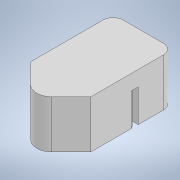
# Autodesk Inventor part: Belt Clip
Saved by Autodesk Inventor 2022 (Build 260153000, 153)
## iProperties
Created: 2022-06-13
Part Number: Belt Clip
Material: Generic
Document SubType Name: Modeling
Designer: Nick
Density: 1 g/cm^3
Appearance: Default
Author: Nick
Autodesk Inventor part; units mm, degrees
ref_plane "YZ Plane" through (0, 0, 0) normal (1, 0, 0) x (0, 1, 0)
ref_plane "XZ Plane" through (0, 0, 0) normal (0, 1, 0) x (-1, 0, 0)
ref_plane "XY Plane" through (0, 0, 0) normal (0, 0, 1) x (1, 0, 0)
sketch "Sketch1" plane through (0, 0, 0) normal (0, 0, 1) x (1, 0, 0)
  line L0 (0, 0) -> (0, 9.5)
  line L1 (0, 9.5) -> (12, 9.5)
  line L2 (12, 9.5) -> (12, 0)
  line L3 (12, 0) -> (7.25, 0)
  line L4 (7.25, 0) -> (7.25, 6.5)
  line L5 (7.25, 6.5) -> (4.75, 6.5)
  line L6 (4.75, 6.5) -> (4.75, 0)
  line L7 (4.75, 0) -> (0, 0)
  line L8 (6, 6.5) -> (6, 0.5) construction
  dimension "d17" = 6.5
  dimension "d18" = 12
  dimension "d20" = 2.5
  dimension "d21" = 3
  constraints: 18 end point, 5 perpendicular, 3 vertical, 2 collinear, 1 horizontal, 1 midpoint
  measures "d17" distance of L5.end L6.end
  measures "d18" distance of L0.end L1.end
  measures "d20" distance of L4.end L5.end
  measures "d21" distance between parallel lines of L5 L1
extrude "Extrusion1" add sketch "Sketch1" along normal blind 7
sketch "Sketch3" plane through (7.25, 0, 0) normal (0, -1, 0) x (1, 0, 0)
  line L0 (-2.5, 0) -> (0, 0) projected
  line L1 (0, 0) -> (0, 7) projected
  line L2 (-2.5, 7) -> (0, 7) projected
  line L3 (-2.5, 0) -> (-2.5, 7) projected
  line L4 (0, 0) -> (4.75, 0) projected
  line L5 (4.75, 0) -> (4.75, 7) projected
  line L6 (0, 7) -> (4.75, 7) projected
  line L7 (0, 0) -> (0, 7) projected
  line L8 (-7.25, 0) -> (-2.5, 0) projected
  line L9 (-2.5, 0) -> (-2.5, 7) projected
  line L10 (-7.25, 7) -> (-2.5, 7) projected
  line L11 (-7.25, 0) -> (-7.25, 7) projected
  line L12 (-7.25, 21.16) -> (4.75, 21.16)
  line L13 (4.75, 21.16) -> (4.75, 8.38)
  line L14 (4.75, 8.38) -> (-7.25, 8.38)
  line L15 (-7.25, 8.38) -> (-7.25, 21.16)
  line L16 (4.75, 8.38) -> (4.25, 7.63)
  line L17 (4.25, 7.63) -> (3.75, 8.38)
  line L18 (4.75, 0) -> (4.75, 7) projected
  line L19 (-7.25, 0) -> (-7.25, 7) projected
  line L20 (-1.25, 8.38) -> (-1.25, 21.16) construction
  line L21 (2.75, 8.38) -> (2.25, 7.63)
  line L22 (2.25, 7.63) -> (1.75, 8.38)
  line L23 (0.75, 8.38) -> (0.25, 7.63)
  line L24 (0.25, 7.63) -> (-0.25, 8.38)
  line L25 (-1.25, 8.38) -> (-1.75, 7.63)
  line L26 (-1.75, 7.63) -> (-2.25, 8.38)
  line L27 (-3.25, 8.38) -> (-3.75, 7.63)
  line L28 (-3.75, 7.63) -> (-4.25, 8.38)
  line L29 (-5.25, 8.38) -> (-5.75, 7.63)
  line L30 (-5.75, 7.63) -> (-6.25, 8.38)
  circle A0 centre (-1.25, 18.16) radius 3
  line L31 (-3.3713, 20.2813) -> (-7.25, 16.4026)
  line L32 (0.8713, 20.2813) -> (4.75, 16.4026)
  point P0 (-6.25, 8.38)
  point P1 (-5.25, 8.38)
  point P2 (-4.25, 8.38)
  point P3 (-3.25, 8.38)
  point P4 (-2.25, 8.38)
  point P5 (-1.25, 8.38)
  point P6 (-0.25, 8.38)
  point P7 (0.75, 8.38)
  point P8 (1.75, 8.38)
  dimension "d22" = 1.38
  dimension "d23" = 12.78
  dimension "d24" = 0.75
  dimension "d25" = 1
  dimension "d28" = 2
  dimension "d42" = 6
  dimension "d43" = 135
  dimension "d44" = 135
  constraints: 38 end point, 3 point on circle, 3 point on line, 3 tangent, 2 collinear, 2 horizontal, 2 midpoint, 2 parallel, 1 centre point, 1 equal length, 1 perpendicular, 25 other
  measures "d22" distance between parallel lines of L6 L14
  measures "d23" distance of L20.start L20.end
  measures "d24" distance from line of L14 L16.end
  measures "d25" distance of L17.end L13.end
  measures "d28" distance of L16.end L21.end
  measures "d42" diameter of A0
  measures "d43" angle of L13 L32
  measures "d44" angle of L15 L31
extrude "Extrusion2" add sketch "Sketch3" against normal up to surface (9.5 mm away) contours A0 | L31 A0 L32 L13 L14 L15 | L14 L29 L30 | L16 L17 L14 | L14 L27 L28 | L21 L22 L14 | L14 L25 L26 | L23 L24 L14
fillet "Fillet2" radius 1 2 edges at (4.75, 3.25, 7) (7.25, 3.25, 7)
fillet "Fillet3" radius 2 4 edges at (12, 4.75, 0) (0, 4.75, 0) (7.25, 3.25, 0) (4.75, 3.25, 0)
chamfer "Chamfer1" distance 0.3 angle 45 6 edges at (11.5, 4.75, 7.63) (9.5, 4.75, 7.63) (7.5, 4.75, 7.63) (5.5, 4.75, 7.63) (3.5, 4.75, 7.63) (1.5, 4.75, 7.63)
sketch "Sketch5" plane through (6, 9.5, 18.16) normal (0, 1, 0) x (1, 0, 0)
  line L0 (-4.6664, 10.2804) -> (-4.3336, 10.2804) projected
  line L1 (-5, 9.78) -> (-4.6664, 10.2804) projected
  line L2 (-6, 9.78) -> (-5, 9.78) projected
  line L3 (-6, 1.7574) -> (-6, 9.78) projected
  line L4 (-2.1213, -2.1213) -> (-6, 1.7574) projected
  arc A0 (-2.1213, -2.1213) -> (2.1213, -2.1213) centre (0, 0) ccw projected
  line L5 (6, 1.7574) -> (2.1213, -2.1213) projected
  line L6 (6, 9.78) -> (6, 1.7574) projected
  line L7 (5.6664, 10.2804) -> (6, 9.78) projected
  line L8 (5.3336, 10.2804) -> (5.6664, 10.2804) projected
  line L9 (5, 9.78) -> (5.3336, 10.2804) projected
  line L10 (4, 9.78) -> (5, 9.78) projected
  line L11 (3.6664, 10.2804) -> (4, 9.78) projected
  line L12 (3.3336, 10.2804) -> (3.6664, 10.2804) projected
  line L13 (3, 9.78) -> (3.3336, 10.2804) projected
  line L14 (2, 9.78) -> (3, 9.78) projected
  line L15 (1.6664, 10.2804) -> (2, 9.78) projected
  line L16 (1.3336, 10.2804) -> (1.6664, 10.2804) projected
  line L17 (1, 9.78) -> (1.3336, 10.2804) projected
  line L18 (0, 9.78) -> (1, 9.78) projected
  line L19 (-0.3336, 10.2804) -> (0, 9.78) projected
  line L20 (-0.6664, 10.2804) -> (-0.3336, 10.2804) projected
  line L21 (-1, 9.78) -> (-0.6664, 10.2804) projected
  line L22 (-2, 9.78) -> (-1, 9.78) projected
  line L23 (-2.3336, 10.2804) -> (-2, 9.78) projected
  line L24 (-2.6664, 10.2804) -> (-2.3336, 10.2804) projected
  line L25 (-3, 9.78) -> (-2.6664, 10.2804) projected
  line L26 (-4, 9.78) -> (-3, 9.78) projected
  line L27 (-4.3336, 10.2804) -> (-4, 9.78) projected
  arc A1 (-4, 18.16) -> (-6, 16.16) centre (-4, 16.16) ccw projected
  line L28 (-6, 16.16) -> (-6, 11.16) projected
  line L29 (6, 11.16) -> (-6, 11.16) projected
  line L30 (6, 16.16) -> (6, 11.16) projected
  arc A2 (6, 16.16) -> (4, 18.16) centre (4, 16.16) ccw projected
  line L31 (4, 18.16) -> (-4, 18.16) projected
  line L32 (-6, 1.7574) -> (-6, 9.78) projected
  line L33 (-6, 9.78) -> (-6, 11.1694)
  line L34 (6, 9.78) -> (6, 11.16)
  point P0 (-6, 18.16)
  constraints: 4 end point, 1 point on line, 1 vertical
extrude "Extrusion4" add sketch "Sketch5" against normal up to surface (3 mm away)
body "Solid1"
